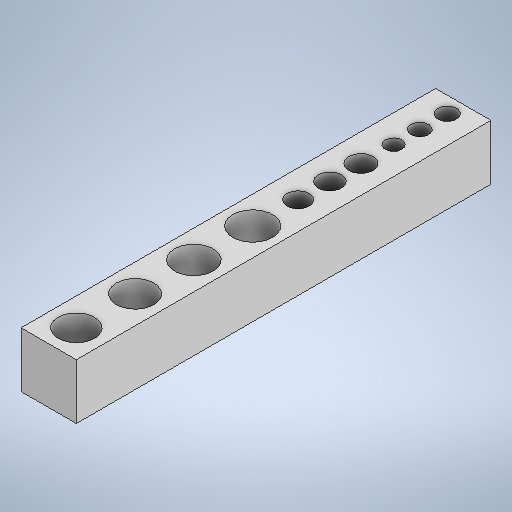
# Autodesk Inventor part: test_print
Saved by Autodesk Inventor 2025.1 (Build 291241000, 241)
## iProperties
Created: 2024-11-19
Part Number: test_print
Material: Ogólny
Document SubType Name: Modeling
Designer: PC
Density: 1 g/cm^3
Appearance: Domyślna
Author: PC
Autodesk Inventor part; units mm, degrees
ref_plane "YZ Plane" through (0, 0, 0) normal (1, 0, 0) x (0, 1, 0)
ref_plane "XZ Plane" through (0, 0, 0) normal (0, 1, 0) x (-1, 0, 0)
ref_plane "XY Plane" through (0, 0, 0) normal (0, 0, 1) x (1, 0, 0)
sketch "Szkic1" plane through (0, 0, 0) normal (0, 1, 0) x (-1, 0, 0)
  line L0 (0, 0) -> (10, 0)
  line L1 (10, 0) -> (10, -75)
  line L2 (10, -75) -> (0, -75)
  line L3 (0, -75) -> (0, 0)
  circle A0 centre (5, -5) radius 3.3
  circle A1 centre (5, -15.6324) radius 3.4
  circle A2 centre (5, -26.2648) radius 3.5
  circle A3 centre (5, -36.8972) radius 3.6
  line L4 (5, -5) -> (5, -15.6324) construction
  line L5 (5, -15.6324) -> (5, -26.2648) construction
  line L6 (5, -26.2648) -> (5, -36.8972) construction
  circle A4 centre (5, -45.1205) radius 2
  circle A5 centre (5, -56.4925) radius 2.2
  circle A6 centre (5, -50.8625) radius 2.1
  circle A7 centre (5, -62.3904) radius 1.5
  circle A8 centre (5, -67.132) radius 1.6
  circle A9 centre (5, -72.0899) radius 1.7
  line L7 (5, -36.8972) -> (5, -75) construction
  dimension "d0" = 10
  dimension "d1" = 75
  dimension "d2" = 6.6
  dimension "d3" = 6.8
  dimension "d4" = 7
  dimension "d5" = 7.2
  dimension "d6" = 5
  dimension "d7" = 4
  dimension "d8" = 4.4
  dimension "d9" = 4.2
  dimension "d12" = 3
  dimension "d13" = 3.2
  dimension "d14" = 3.4
  constraints: 16 end point, 10 centre point, 4 equal length, 3 point on line, 2 collinear, 1 horizontal, 1 midpoint, 1 perpendicular, 1 vertical
  measures "d0" distance of L1.end L2.end
  measures "d1" distance of L0.end L1.end
  measures "d2" diameter of A0
  measures "d3" diameter of A1
  measures "d4" diameter of A2
  measures "d5" diameter of A3
  measures "d6" distance from line of L0 L4.start
  measures "d7" diameter of A4
  measures "d8" diameter of A5
  measures "d9" diameter of A6
  measures "d12" diameter of A7
  measures "d13" diameter of A8
  measures "d14" diameter of A9
extrude "Wyciągnięcie proste1" add sketch "Szkic1" along normal blind 10
